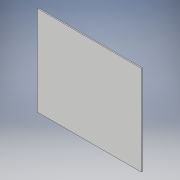
# Autodesk Inventor part: Part1
Saved by Autodesk Inventor 2018 (Build 220112000, 112)
## iProperties
Created: 2020-02-11
Part Number: Part1
Material: Generic
Document SubType Name: Modeling
Designer: Sam
Density: 1 g/cm^3
Appearance: Default
Author: Sam
Autodesk Inventor part; units mm, degrees
ref_plane "YZ Plane" through (0, 0, 0) normal (1, 0, 0) x (0, 1, 0)
ref_plane "XZ Plane" through (0, 0, 0) normal (0, 1, 0) x (-1, 0, 0)
ref_plane "XY Plane" through (0, 0, 0) normal (0, 0, 1) x (1, 0, 0)
sketch "Sketch1" plane through (0, 0, 0) normal (0, 0, 1) x (1, 0, 0)
  line L0 (76.2, -65.8876) -> (-76.2, -65.8876)
  line L1 (-76.2, -65.8876) -> (-76.2, 65.8876)
  line L2 (-76.2, 65.8876) -> (76.2, 65.8876)
  line L3 (76.2, 65.8876) -> (76.2, -65.8876)
  line L4 (76.2, -65.8876) -> (-76.2, 65.8876) construction
  line L5 (-76.2, -65.8876) -> (76.2, 65.8876) construction
  line L6 (-76.2, -65.8876) -> (-57.6516, -65.8876)
  line L7 (76.2, -65.8876) -> (57.6517, -65.8876)
  point P0 (0, 0)
  dimension "d10" = 131.7752
  dimension "d11" = 152.4
  constraints: 16 end point, 2 midpoint, 2 parallel, 2 point on line, 1 horizontal, 1 perpendicular
  measures "d10" distance of L0.end L1.end
  measures "d11" distance of L1.end L2.end
extrude "Extrusion2" add sketch "Sketch1" along normal blind 1.5875
body "Solid2"
